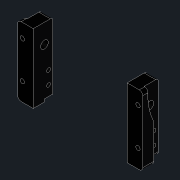
# Autodesk Inventor part: base44
Saved by Autodesk Inventor 2022 (Build 260153000, 153)
## iProperties
Created: 2021-08-30
Part Number: base44
Material: ABS プラスチック
Document SubType Name: Modeling
Designer: Yuta Kage
Density: 1.06 g/cm^3
Appearance: 滑らか - 黒
Author: Yuta Kage
Autodesk Inventor part; units mm, degrees
ref_plane "XZ Plane" through (0, 0, 0) normal (0, 1, 0) x (-1, 0, 0)
ref_plane "XY Plane" through (0, 0, 0) normal (0, 0, 1) x (1, 0, 0)
sketch "スケッチ2" plane through (0, 0, 0) normal (0, 0, 1) x (1, 0, 0)
  line L0 (-70.25, -25) -> (70.25, -25) construction
  line L1 (70.25, -25) -> (70.25, 50) construction
  line L2 (70.25, 50) -> (-70.25, 50) construction
  line L3 (-70.25, 50) -> (-70.25, -25) construction
  line L4 (73.25, -28) -> (-73.25, -28)
  line L5 (-73.25, -28) -> (-73.25, 53)
  line L6 (-73.25, 53) -> (73.25, 53)
  line L7 (73.25, 53) -> (73.25, -28)
  point P0 (0, 0)
  dimension "d0" = 140.5
  dimension "d2" = 3
  dimension "d3" = 3
  dimension "d58" = 50
  dimension "d59" = 3
  dimension "d60" = 25
  dimension "d72" = 3
  dimension "d73" = 70.25
  constraints: 16 end point, 4 parallel, 2 horizontal, 2 perpendicular
  measures "d0" distance of L2.end L1.end
  measures "d2" distance between parallel lines of L2 L6
  measures "d3" distance between parallel lines of L5 L3
  measures "d58" distance from line of point (0, 0) L2
  measures "d59" distance between parallel lines of L7 L1
  measures "d60" distance from line of L0 point (0, 0)
  measures "d72" distance between parallel lines of L4 L0
  measures "d73" distance from line of point (0, 0) L3
extrude "押し出し1" add sketch "スケッチ2" along normal blind 23
ref_plane "作業平面1" through (68.5, 0, 0) normal (1, 0, 0) x (0, 1, 0)
sketch "スケッチ3" plane through (68.5, -28, 0) normal (1, 0, 0) x (0, 0, -1)
  circle A0 centre (50.5, 74.5) radius 67.5
  line L0 (0, 0) -> (-23, 0) projected
  line L1 (0, 0) -> (0, 81) projected
  line L2 (-10, 44.5667) -> (-10, 0)
  line L3 (0, 0) -> (-23, 0) projected
  point P0 (0, 28)
  point P1 (0, 29.7116)
  dimension "d6" = 135
  dimension "d7" = 74.5
  dimension "d9" = 60.5
  dimension "d23" = 10
  constraints: 2 end point, 1 perpendicular, 1 point on line, 3 other
  measures "d7" distance from line of point (50.5, 74.5) L0
  measures "d9" distance from line of point (50.5, 74.5) L2
  measures "d23" distance between parallel lines of L2 L1
extrude "押し出し2" cut sketch "スケッチ3" along normal through all
sketch "スケッチ4" plane through (0, 0, 23) normal (0, 0, 1) x (1, 0, 0)
  line L0 (-67.75, -6.75) -> (67.75, -6.75)
  line L1 (67.75, -6.75) -> (67.75, 36.75)
  line L2 (67.75, 36.75) -> (-67.75, 36.75)
  line L3 (-67.75, 36.75) -> (-67.75, -6.75)
  line L4 (-67.75, -6.75) -> (67.75, 36.75) construction
  line L5 (67.75, -6.75) -> (-67.75, 36.75) construction
  line L6 (73.25, 53) -> (-73.25, 53) projected
  point P0 (0, 0)
  point P1 (0, 15)
  dimension "d13" = 135.5
  dimension "d14" = 43.5
  dimension "d86" = 15
  constraints: 12 end point, 2 parallel, 1 horizontal, 1 midpoint, 1 perpendicular, 1 vertical alignment
  measures "d13" distance of L2.end L1.end
  measures "d14" distance of L1.end L0.end
  measures "d86" distance of point (0, 0) point (0, 15)
hole "穴1" at (67.75, -6.75, 23) at (67.75, 36.75, 23) at (-67.75, 36.75, 23) at (-67.75, -6.75, 23) direction (0, 0, -1) diameter 5 depth 6 tip angle 118
sketch "スケッチ5" plane through (68.5, -28, 0) normal (1, 0, 0) x (0, 0, -1)
  line L0 (0, 0) -> (-10, 0) projected
  line L1 (-10, 0) -> (-10, 44.5667) projected
  point P0 (0, 28)
  point P1 (-5, 15)
  point P2 (-5, 30)
  point P3 (-10, 35.913)
  dimension "d24" = 15
  dimension "d25" = 15
  dimension "d26" = 5
  constraints: 1 vertical alignment
  measures "d24" distance from line of L0 point (-5, 15)
  measures "d25" distance of point (-5, 15) point (-5, 30)
  measures "d26" distance from line of L1 point (-5, 15)
hole "穴2" at (68.5, -13, 5) at (68.5, 2, 5) direction (-1, 0, 0) diameter 4.5 end through all clearance for "Flat Head Machine Screw" size "M4" standard "Ansi Metric M Profile"
fillet "フィレット2" radius 10 1 edges at (70.875, 16.5667, 10)
sketch "スケッチ11" plane through (-73.25, 53, 23) normal (0, 1, 0) x (1, 0, 0)
  line L0 (0, 23) -> (141.75, 23) projected
  line L1 (0, 0) -> (146.5, 0) projected
  line L2 (18.25, 0) -> (128.25, 0)
  line L3 (128.25, 0) -> (128.25, 23)
  line L4 (128.25, 23) -> (18.25, 23)
  line L5 (18.25, 23) -> (18.25, 0)
  line L6 (141.75, 6.3137) -> (141.75, 23) projected
  line L7 (146.5, 6.3137) -> (146.5, 0) projected
  line L8 (0, 23) -> (0, 0) projected
  dimension "d68" = 18.25
  dimension "d69" = 18.25
  dimension "d70" = 0
  constraints: 8 end point, 2 parallel, 1 horizontal, 1 perpendicular, 1 point on line
  measures "d68" distance between parallel lines of L8 L5
  measures "d69" distance between parallel lines of L7 L3
  measures "d70" distance between parallel lines of L0 L4
extrude "押し出し8" cut sketch "スケッチ11" against normal through all contours L0 L3 L1 L5
mirror "ミラー1" about plane through (0, 0, 0) normal (1, 0, 0) of "押し出し2", "穴2", "フィレット2"
sketch "スケッチ7" plane through (0, 0, 0) normal (0, 0, -1) x (-1, 0, 0)
  line L0 (68.5, -28) -> (68.5, 53) projected
  line L1 (-68.5, -24.8) -> (68.5, -24.8)
  line L2 (68.5, -24.8) -> (68.5, -28)
  line L3 (68.5, -28) -> (-68.5, -28)
  line L4 (-68.5, -28) -> (-68.5, -24.8)
  line L5 (-68.5, -24.8) -> (68.5, -28) construction
  line L6 (68.5, -24.8) -> (-68.5, -28) construction
  point P0 (0, 0)
  point P1 (0, -26.4)
  point P2 (-68.5, -28)
  point P3 (68.5, -24.8)
  dimension "d38" = 3.2
  constraints: 12 end point, 2 midpoint, 2 parallel, 1 coincident, 1 horizontal, 1 perpendicular
  measures "d38" distance of L3.end L1.start
extrude "押し出し4" cut sketch "スケッチ7" against normal up to surface (10 mm away)
fillet "フィレット3" radius 3.2 2 edges at (68.5, -24.8, 5) (-68.5, -24.8, 5)
fillet "フィレット6" radius 4 4 edges at (73.25, -28, 16.5) (-73.25, -28, 16.5) (73.25, 53, 19.8432) (-73.25, 53, 19.8432)
fillet "フィレット8" radius 3 2 edges at (-61.75, 53, 0) (61.75, 53, 0)
sketch "スケッチ12" plane through (68.5, -28, 0) normal (1, 0, 0) x (0, 0, -1)
  circle A0 centre (50.5, 74.5) radius 67.5 projected
  circle A1 centre (50.5, 74.5) radius 62.5
  line L0 (-9.8704, 58.3238) -> (50.5, 74.5)
  line L1 (-16.6863, 81) -> (-3, 81) projected
  point P0 (0, 28)
  dimension "d75" = 125
  dimension "d76" = 15
  constraints: 2 end point, 1 coincident, 4 other
  measures "d76" angle of L1 L0
hole "穴3" at (68.5, 30.3238, 9.8704) direction (-1, 0, 0) diameter 9 end through all
equation "\"d2\" = d3"
equation "\"d69\" = d68"
